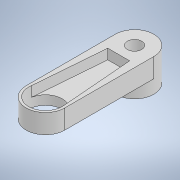
# Autodesk Inventor part: Поворотный рычаг для сервы
Saved by Autodesk Inventor 2020 (Build 240168000, 168)
## iProperties
Created: 2021-04-11
Part Number: Поворотный рычаг для сервы
Material: Типовые
Document SubType Name: Modeling
Designer: Антон
Density: 1 g/cm^3
Appearance: По умолчанию
Author: Антон
Autodesk Inventor part; units mm, degrees
ref_plane "YZ Plane" through (0, 0, 0) normal (1, 0, 0) x (0, 1, 0)
ref_plane "XZ Plane" through (0, 0, 0) normal (0, 1, 0) x (-1, 0, 0)
ref_plane "XY Plane" through (0, 0, 0) normal (0, 0, 1) x (1, 0, 0)
sketch "Эскиз1" plane through (0, 0, 0) normal (0, 1, 0) x (-1, 0, 0)
  circle A0 centre (0, 0) radius 4
  dimension "d0" = 8
  constraints: 1 centre point, 1 coincident
  measures "d0" diameter of A0
extrude "Выдавливание1" add sketch "Эскиз1" along normal blind 4
sketch "Эскиз5" plane through (0, 4, 0) normal (0, 1, 0) x (1, 0, 0)
  circle A0 centre (0, 0) radius 4 projected
  line L0 (-4, 0) -> (4, 0)
  line L1 (4, 0) -> (4, 18.5)
  line L2 (4, 18.5) -> (-4, 18.5)
  line L3 (-4, 18.5) -> (-4, 0)
  circle A1 centre (0, 0) radius 4 projected
  point P0 (4, 0)
  dimension "d27" = 18.5
  constraints: 8 end point, 2 parallel, 1 coincident, 1 horizontal, 1 midpoint, 1 perpendicular, 1 point on circle, 2 other
  measures "d27" distance of L1.end L0.end
extrude "Выдавливание4" add sketch "Эскиз5" against normal blind 4 contours A0 L3 L2 L1
sketch "Эскиз9" plane through (0, 4, 0) normal (0, -1, 0) x (1, 0, 0)
  circle A0 centre (0, 0) radius 3.5
  line L0 (3.5, 0) -> (-3.5, 0)
  line L1 (3.5, 0) -> (2.25, -15.5)
  line L2 (-3.5, 0) -> (-2.25, -15.5)
  line L3 (2.25, -15.5) -> (-2.25, -15.5)
  point P0 (0, -15.5)
  point P1 (-3.4548, -0.5609)
  point P2 (3.4548, -0.5609)
  dimension "d43" = 7
  dimension "d44" = 4.5
  dimension "d45" = 15.5
  constraints: 8 end point, 2 coincident, 2 horizontal, 2 midpoint, 2 point on circle, 1 centre point, 1 equal length, 1 vertical alignment
  measures "d43" diameter of A0
  measures "d44" distance of L1.end L2.end
  measures "d45" distance from line of L3 point (0, 0)
extrude "Выдавливание7" cut sketch "Эскиз9" along normal blind 2.1
sketch "Эскиз10" plane through (0, 1.9, 0) normal (0, 1, 0) x (1, 0, 0)
  line L0 (2.25, 15.5) -> (3.4548, 0.5609) projected
  line L1 (-2.25, 15.5) -> (2.25, 15.5) projected
  line L2 (-3.4548, 0.5609) -> (-2.25, 15.5) projected
  arc A0 (-3.4548, 0.5609) -> (3.4548, 0.5609) centre (0, 0) ccw projected
  arc A1 (-3.4548, 0.5609) -> (3.4548, 0.5609) centre (0, 0) ccw projected
  circle A2 centre (0, 0) radius 3.5
  point P0 (3.4548, 0.5609)
  constraints: 1 coincident, 3 other
extrude "Выдавливание8" cut sketch "Эскиз10" against normal through all contours A0 A2
sketch "Эскиз6" plane through (0, 4, 0) normal (0, 1, 0) x (1, 0, 0)
  line L0 (-4, 18.5) -> (4, 18.5) projected
  circle A0 centre (0, 18.5) radius 4
  point P0 (0, 0)
  dimension "d30" = 8
  constraints: 1 centre point, 1 midpoint
  measures "d30" diameter of A0
extrude "Выдавливание5" add sketch "Эскиз6" against normal blind 6.8
sketch "Эскиз7" plane through (0, -2.8, -18.5) normal (0, -1, 0) x (1, 0, 0)
  arc A0 (-4, 0) -> (4, 0) centre (0, 0) ccw projected
  arc A1 (4, 0) -> (-4, 0) centre (0, 0) ccw projected
  circle A2 centre (0, 0) radius 2.5
  point P0 (0, 18.5)
  point P1 (3.35, -2.1857)
  point P2 (-3.35, -2.1857)
  dimension "d33" = 5
  constraints: 1 centre point, 1 coincident
  measures "d33" diameter of A2
extrude "Выдавливание6" cut sketch "Эскиз7" against normal blind 2.5 contours A2
sketch "Эскиз8" plane through (0, 4, 0) normal (0, 1, 0) x (1, 0, 0)
  circle A0 centre (0, 18.5) radius 2.5 projected
  point P0 (0, 0)
hole "Отверстие2" at (0, 4, -18.5) direction (0, -1, 0) diameter 3 end through all
sketch "Эскиз11" plane through (0, 4, 0) normal (0, 1, 0) x (1, 0, 0)
  line L0 (-3.4548, 0.5609) -> (-2.2735, 15.2089) projected
  line L1 (2.2735, 15.2089) -> (3.4548, 0.5609) projected
  line L2 (-2.2735, 15.2089) -> (2.2735, 15.2089)
  arc A0 (-2.2735, 15.2089) -> (2.2735, 15.2089) centre (0, 18.5) ccw projected
  line L3 (-3.4548, 0.5609) -> (-2.2735, 15.2089) projected
  arc A1 (3.4548, 0.5609) -> (-3.4548, 0.5609) centre (0, 0) ccw projected
  line L4 (2.2735, 15.2089) -> (3.4548, 0.5609) projected
  constraints: 2 end point, 1 horizontal
extrude "Выдавливание9" cut sketch "Эскиз11" against normal up to surface (2.1 mm away)
